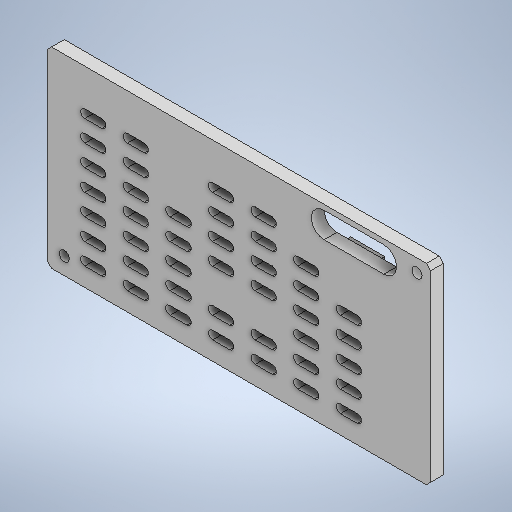
# Autodesk Inventor part: tampa final
Saved by Autodesk Inventor 2025 (Build 290162000, 162)
## iProperties
Created: 2026-04-08
Part Number: tampa final
Material: Genérico
Document SubType Name: Modeling
Designer: pedro
Density: 1 g/cm^3
Appearance: Padrão
Author: pedro
Autodesk Inventor part; units mm, degrees
ref_plane "YZ Plane" through (0, 0, 0) normal (1, 0, 0) x (0, 1, 0)
ref_plane "XZ Plane" through (0, 0, 0) normal (0, 1, 0) x (-1, 0, 0)
ref_plane "XY Plane" through (0, 0, 0) normal (0, 0, 1) x (1, 0, 0)
sketch "Esboço1" plane through (0, 0, 0) normal (0, 0, 1) x (1, 0, 0)
  line L0 (0, 0) -> (90, 0)
  line L1 (90, 0) -> (90, 45)
  line L2 (90, 45) -> (0, 45)
  line L3 (0, 45) -> (0, 0)
  dimension "d0" = 90
  dimension "d1" = 45
  constraints: 8 end point, 2 parallel, 1 horizontal, 1 perpendicular
  measures "d0" distance of L2.end L1.end
  measures "d1" distance of L1.end L0.end
extrude "Extrusão1" add sketch "Esboço1" along normal blind 3
sketch "Esboço3" plane through (0, 0, 3) normal (0, 0, 1) x (1, 0, 0)
  line L0 (0, 45) -> (0, 0) projected
  line L1 (90, 45) -> (0, 45) projected
  line L2 (63.8381, 29.7994) -> (75.2312, 29.7994)
  line L3 (8.8095, 35.3501) -> (12.8095, 35.3501) construction
  line L4 (8.8095, 34.3501) -> (12.8095, 34.3501)
  line L5 (12.8095, 36.3501) -> (8.8095, 36.3501)
  arc A0 (8.8095, 36.3501) -> (8.8095, 34.3501) centre (8.8095, 35.3501) ccw
  arc A1 (12.8095, 34.3501) -> (12.8095, 36.3501) centre (12.8095, 35.3501) ccw
  arc A2 (22.8095, 34.3501) -> (22.8095, 36.3501) centre (22.8095, 35.3501) ccw
  line L6 (18.8095, 35.3501) -> (22.8095, 35.3501) construction
  line L7 (18.8095, 34.3501) -> (22.8095, 34.3501)
  line L8 (22.8095, 36.3501) -> (18.8095, 36.3501)
  arc A3 (18.8095, 36.3501) -> (18.8095, 34.3501) centre (18.8095, 35.3501) ccw
  arc A4 (32.8095, 34.3501) -> (32.8095, 36.3501) centre (32.8095, 35.3501) ccw
  line L9 (28.8095, 35.3501) -> (32.8095, 35.3501) construction
  line L10 (28.8095, 34.3501) -> (32.8095, 34.3501)
  line L11 (32.8095, 36.3501) -> (28.8095, 36.3501)
  arc A5 (28.8095, 36.3501) -> (28.8095, 34.3501) centre (28.8095, 35.3501) ccw
  arc A6 (42.8095, 34.3501) -> (42.8095, 36.3501) centre (42.8095, 35.3501) ccw
  line L12 (38.8095, 35.3501) -> (42.8095, 35.3501) construction
  line L13 (38.8095, 34.3501) -> (42.8095, 34.3501)
  line L14 (42.8095, 36.3501) -> (38.8095, 36.3501)
  arc A7 (38.8095, 36.3501) -> (38.8095, 34.3501) centre (38.8095, 35.3501) ccw
  arc A8 (52.8095, 34.3501) -> (52.8095, 36.3501) centre (52.8095, 35.3501) ccw
  line L15 (48.8095, 35.3501) -> (52.8095, 35.3501) construction
  line L16 (48.8095, 34.3501) -> (52.8095, 34.3501)
  line L17 (52.8095, 36.3501) -> (48.8095, 36.3501)
  arc A9 (48.8095, 36.3501) -> (48.8095, 34.3501) centre (48.8095, 35.3501) ccw
  arc A10 (12.8095, 29.3501) -> (12.8095, 31.3501) centre (12.8095, 30.3501) ccw
  line L18 (8.8095, 30.3501) -> (12.8095, 30.3501) construction
  line L19 (8.8095, 29.3501) -> (12.8095, 29.3501)
  line L20 (12.8095, 31.3501) -> (8.8095, 31.3501)
  arc A11 (8.8095, 31.3501) -> (8.8095, 29.3501) centre (8.8095, 30.3501) ccw
  arc A12 (22.8095, 29.3501) -> (22.8095, 31.3501) centre (22.8095, 30.3501) ccw
  line L21 (18.8095, 30.3501) -> (22.8095, 30.3501) construction
  line L22 (18.8095, 29.3501) -> (22.8095, 29.3501)
  line L23 (22.8095, 31.3501) -> (18.8095, 31.3501)
  arc A13 (18.8095, 31.3501) -> (18.8095, 29.3501) centre (18.8095, 30.3501) ccw
  arc A14 (32.8095, 29.3501) -> (32.8095, 31.3501) centre (32.8095, 30.3501) ccw
  line L24 (28.8095, 30.3501) -> (32.8095, 30.3501) construction
  line L25 (28.8095, 29.3501) -> (32.8095, 29.3501)
  line L26 (32.8095, 31.3501) -> (28.8095, 31.3501)
  arc A15 (28.8095, 31.3501) -> (28.8095, 29.3501) centre (28.8095, 30.3501) ccw
  arc A16 (42.8095, 29.3501) -> (42.8095, 31.3501) centre (42.8095, 30.3501) ccw
  line L27 (38.8095, 30.3501) -> (42.8095, 30.3501) construction
  line L28 (38.8095, 29.3501) -> (42.8095, 29.3501)
  line L29 (42.8095, 31.3501) -> (38.8095, 31.3501)
  arc A17 (38.8095, 31.3501) -> (38.8095, 29.3501) centre (38.8095, 30.3501) ccw
  arc A18 (52.8095, 29.3501) -> (52.8095, 31.3501) centre (52.8095, 30.3501) ccw
  line L30 (48.8095, 30.3501) -> (52.8095, 30.3501) construction
  line L31 (48.8095, 29.3501) -> (52.8095, 29.3501)
  line L32 (52.8095, 31.3501) -> (48.8095, 31.3501)
  arc A19 (48.8095, 31.3501) -> (48.8095, 29.3501) centre (48.8095, 30.3501) ccw
  arc A20 (62.8095, 29.3501) -> (62.8095, 31.3501) centre (62.8095, 30.3501) ccw
  line L33 (58.8095, 30.3501) -> (62.8095, 30.3501) construction
  line L34 (58.8095, 29.3501) -> (62.8095, 29.3501)
  line L35 (62.8095, 31.3501) -> (58.8095, 31.3501)
  arc A21 (58.8095, 31.3501) -> (58.8095, 29.3501) centre (58.8095, 30.3501) ccw
  arc A22 (72.8095, 29.3501) -> (72.8095, 31.3501) centre (72.8095, 30.3501) ccw
  line L36 (68.8095, 30.3501) -> (72.8095, 30.3501) construction
  line L37 (68.8095, 29.3501) -> (72.8095, 29.3501)
  line L38 (72.8095, 31.3501) -> (68.8095, 31.3501)
  arc A23 (68.8095, 31.3501) -> (68.8095, 29.3501) centre (68.8095, 30.3501) ccw
  arc A24 (12.8095, 24.3501) -> (12.8095, 26.3501) centre (12.8095, 25.3501) ccw
  line L39 (8.8095, 25.3501) -> (12.8095, 25.3501) construction
  line L40 (8.8095, 24.3501) -> (12.8095, 24.3501)
  line L41 (12.8095, 26.3501) -> (8.8095, 26.3501)
  arc A25 (8.8095, 26.3501) -> (8.8095, 24.3501) centre (8.8095, 25.3501) ccw
  arc A26 (22.8095, 24.3501) -> (22.8095, 26.3501) centre (22.8095, 25.3501) ccw
  line L42 (18.8095, 25.3501) -> (22.8095, 25.3501) construction
  line L43 (18.8095, 24.3501) -> (22.8095, 24.3501)
  line L44 (22.8095, 26.3501) -> (18.8095, 26.3501)
  arc A27 (18.8095, 26.3501) -> (18.8095, 24.3501) centre (18.8095, 25.3501) ccw
  arc A28 (32.8095, 24.3501) -> (32.8095, 26.3501) centre (32.8095, 25.3501) ccw
  line L45 (28.8095, 25.3501) -> (32.8095, 25.3501) construction
  line L46 (28.8095, 24.3501) -> (32.8095, 24.3501)
  line L47 (32.8095, 26.3501) -> (28.8095, 26.3501)
  arc A29 (28.8095, 26.3501) -> (28.8095, 24.3501) centre (28.8095, 25.3501) ccw
  arc A30 (42.8095, 24.3501) -> (42.8095, 26.3501) centre (42.8095, 25.3501) ccw
  line L48 (38.8095, 25.3501) -> (42.8095, 25.3501) construction
  line L49 (38.8095, 24.3501) -> (42.8095, 24.3501)
  line L50 (42.8095, 26.3501) -> (38.8095, 26.3501)
  arc A31 (38.8095, 26.3501) -> (38.8095, 24.3501) centre (38.8095, 25.3501) ccw
  arc A32 (52.8095, 24.3501) -> (52.8095, 26.3501) centre (52.8095, 25.3501) ccw
  line L51 (48.8095, 25.3501) -> (52.8095, 25.3501) construction
  line L52 (48.8095, 24.3501) -> (52.8095, 24.3501)
  line L53 (52.8095, 26.3501) -> (48.8095, 26.3501)
  arc A33 (48.8095, 26.3501) -> (48.8095, 24.3501) centre (48.8095, 25.3501) ccw
  arc A34 (62.8095, 24.3501) -> (62.8095, 26.3501) centre (62.8095, 25.3501) ccw
  line L54 (58.8095, 25.3501) -> (62.8095, 25.3501) construction
  line L55 (58.8095, 24.3501) -> (62.8095, 24.3501)
  line L56 (62.8095, 26.3501) -> (58.8095, 26.3501)
  arc A35 (58.8095, 26.3501) -> (58.8095, 24.3501) centre (58.8095, 25.3501) ccw
  arc A36 (72.8095, 24.3501) -> (72.8095, 26.3501) centre (72.8095, 25.3501) ccw
  line L57 (68.8095, 25.3501) -> (72.8095, 25.3501) construction
  line L58 (68.8095, 24.3501) -> (72.8095, 24.3501)
  line L59 (72.8095, 26.3501) -> (68.8095, 26.3501)
  arc A37 (68.8095, 26.3501) -> (68.8095, 24.3501) centre (68.8095, 25.3501) ccw
  arc A38 (12.8095, 19.3501) -> (12.8095, 21.3501) centre (12.8095, 20.3501) ccw
  line L60 (8.8095, 20.3501) -> (12.8095, 20.3501) construction
  line L61 (8.8095, 19.3501) -> (12.8095, 19.3501)
  line L62 (12.8095, 21.3501) -> (8.8095, 21.3501)
  arc A39 (8.8095, 21.3501) -> (8.8095, 19.3501) centre (8.8095, 20.3501) ccw
  arc A40 (22.8095, 19.3501) -> (22.8095, 21.3501) centre (22.8095, 20.3501) ccw
  line L63 (18.8095, 20.3501) -> (22.8095, 20.3501) construction
  line L64 (18.8095, 19.3501) -> (22.8095, 19.3501)
  line L65 (22.8095, 21.3501) -> (18.8095, 21.3501)
  arc A41 (18.8095, 21.3501) -> (18.8095, 19.3501) centre (18.8095, 20.3501) ccw
  arc A42 (32.8095, 19.3501) -> (32.8095, 21.3501) centre (32.8095, 20.3501) ccw
  line L66 (28.8095, 20.3501) -> (32.8095, 20.3501) construction
  line L67 (28.8095, 19.3501) -> (32.8095, 19.3501)
  line L68 (32.8095, 21.3501) -> (28.8095, 21.3501)
  arc A43 (28.8095, 21.3501) -> (28.8095, 19.3501) centre (28.8095, 20.3501) ccw
  arc A44 (42.8095, 19.3501) -> (42.8095, 21.3501) centre (42.8095, 20.3501) ccw
  line L69 (38.8095, 20.3501) -> (42.8095, 20.3501) construction
  line L70 (38.8095, 19.3501) -> (42.8095, 19.3501)
  line L71 (42.8095, 21.3501) -> (38.8095, 21.3501)
  arc A45 (38.8095, 21.3501) -> (38.8095, 19.3501) centre (38.8095, 20.3501) ccw
  arc A46 (52.8095, 19.3501) -> (52.8095, 21.3501) centre (52.8095, 20.3501) ccw
  line L72 (48.8095, 20.3501) -> (52.8095, 20.3501) construction
  line L73 (48.8095, 19.3501) -> (52.8095, 19.3501)
  line L74 (52.8095, 21.3501) -> (48.8095, 21.3501)
  arc A47 (48.8095, 21.3501) -> (48.8095, 19.3501) centre (48.8095, 20.3501) ccw
  arc A48 (62.8095, 19.3501) -> (62.8095, 21.3501) centre (62.8095, 20.3501) ccw
  line L75 (58.8095, 20.3501) -> (62.8095, 20.3501) construction
  line L76 (58.8095, 19.3501) -> (62.8095, 19.3501)
  line L77 (62.8095, 21.3501) -> (58.8095, 21.3501)
  arc A49 (58.8095, 21.3501) -> (58.8095, 19.3501) centre (58.8095, 20.3501) ccw
  arc A50 (72.8095, 19.3501) -> (72.8095, 21.3501) centre (72.8095, 20.3501) ccw
  line L78 (68.8095, 20.3501) -> (72.8095, 20.3501) construction
  line L79 (68.8095, 19.3501) -> (72.8095, 19.3501)
  line L80 (72.8095, 21.3501) -> (68.8095, 21.3501)
  arc A51 (68.8095, 21.3501) -> (68.8095, 19.3501) centre (68.8095, 20.3501) ccw
  arc A52 (12.8095, 14.3501) -> (12.8095, 16.3501) centre (12.8095, 15.3501) ccw
  line L81 (8.8095, 15.3501) -> (12.8095, 15.3501) construction
  line L82 (8.8095, 14.3501) -> (12.8095, 14.3501)
  line L83 (12.8095, 16.3501) -> (8.8095, 16.3501)
  arc A53 (8.8095, 16.3501) -> (8.8095, 14.3501) centre (8.8095, 15.3501) ccw
  arc A54 (22.8095, 14.3501) -> (22.8095, 16.3501) centre (22.8095, 15.3501) ccw
  line L84 (18.8095, 15.3501) -> (22.8095, 15.3501) construction
  line L85 (18.8095, 14.3501) -> (22.8095, 14.3501)
  line L86 (22.8095, 16.3501) -> (18.8095, 16.3501)
  arc A55 (18.8095, 16.3501) -> (18.8095, 14.3501) centre (18.8095, 15.3501) ccw
  arc A56 (32.8095, 14.3501) -> (32.8095, 16.3501) centre (32.8095, 15.3501) ccw
  line L87 (28.8095, 15.3501) -> (32.8095, 15.3501) construction
  line L88 (28.8095, 14.3501) -> (32.8095, 14.3501)
  line L89 (32.8095, 16.3501) -> (28.8095, 16.3501)
  arc A57 (28.8095, 16.3501) -> (28.8095, 14.3501) centre (28.8095, 15.3501) ccw
  arc A58 (42.8095, 14.3501) -> (42.8095, 16.3501) centre (42.8095, 15.3501) ccw
  line L90 (38.8095, 15.3501) -> (42.8095, 15.3501) construction
  line L91 (38.8095, 14.3501) -> (42.8095, 14.3501)
  line L92 (42.8095, 16.3501) -> (38.8095, 16.3501)
  arc A59 (38.8095, 16.3501) -> (38.8095, 14.3501) centre (38.8095, 15.3501) ccw
  arc A60 (52.8095, 14.3501) -> (52.8095, 16.3501) centre (52.8095, 15.3501) ccw
  line L93 (48.8095, 15.3501) -> (52.8095, 15.3501) construction
  line L94 (48.8095, 14.3501) -> (52.8095, 14.3501)
  line L95 (52.8095, 16.3501) -> (48.8095, 16.3501)
  arc A61 (48.8095, 16.3501) -> (48.8095, 14.3501) centre (48.8095, 15.3501) ccw
  arc A62 (62.8095, 14.3501) -> (62.8095, 16.3501) centre (62.8095, 15.3501) ccw
  line L96 (58.8095, 15.3501) -> (62.8095, 15.3501) construction
  line L97 (58.8095, 14.3501) -> (62.8095, 14.3501)
  line L98 (62.8095, 16.3501) -> (58.8095, 16.3501)
  arc A63 (58.8095, 16.3501) -> (58.8095, 14.3501) centre (58.8095, 15.3501) ccw
  arc A64 (72.8095, 14.3501) -> (72.8095, 16.3501) centre (72.8095, 15.3501) ccw
  line L99 (68.8095, 15.3501) -> (72.8095, 15.3501) construction
  line L100 (68.8095, 14.3501) -> (72.8095, 14.3501)
  line L101 (72.8095, 16.3501) -> (68.8095, 16.3501)
  arc A65 (68.8095, 16.3501) -> (68.8095, 14.3501) centre (68.8095, 15.3501) ccw
  arc A66 (12.8095, 9.3501) -> (12.8095, 11.3501) centre (12.8095, 10.3501) ccw
  line L102 (8.8095, 10.3501) -> (12.8095, 10.3501) construction
  line L103 (8.8095, 9.3501) -> (12.8095, 9.3501)
  line L104 (12.8095, 11.3501) -> (8.8095, 11.3501)
  arc A67 (8.8095, 11.3501) -> (8.8095, 9.3501) centre (8.8095, 10.3501) ccw
  arc A68 (22.8095, 9.3501) -> (22.8095, 11.3501) centre (22.8095, 10.3501) ccw
  line L105 (18.8095, 10.3501) -> (22.8095, 10.3501) construction
  line L106 (18.8095, 9.3501) -> (22.8095, 9.3501)
  line L107 (22.8095, 11.3501) -> (18.8095, 11.3501)
  arc A69 (18.8095, 11.3501) -> (18.8095, 9.3501) centre (18.8095, 10.3501) ccw
  arc A70 (32.8095, 9.3501) -> (32.8095, 11.3501) centre (32.8095, 10.3501) ccw
  line L108 (28.8095, 10.3501) -> (32.8095, 10.3501) construction
  line L109 (28.8095, 9.3501) -> (32.8095, 9.3501)
  line L110 (32.8095, 11.3501) -> (28.8095, 11.3501)
  arc A71 (28.8095, 11.3501) -> (28.8095, 9.3501) centre (28.8095, 10.3501) ccw
  arc A72 (42.8095, 9.3501) -> (42.8095, 11.3501) centre (42.8095, 10.3501) ccw
  line L111 (38.8095, 10.3501) -> (42.8095, 10.3501) construction
  line L112 (38.8095, 9.3501) -> (42.8095, 9.3501)
  line L113 (42.8095, 11.3501) -> (38.8095, 11.3501)
  arc A73 (38.8095, 11.3501) -> (38.8095, 9.3501) centre (38.8095, 10.3501) ccw
  arc A74 (52.8095, 9.3501) -> (52.8095, 11.3501) centre (52.8095, 10.3501) ccw
  line L114 (48.8095, 10.3501) -> (52.8095, 10.3501) construction
  line L115 (48.8095, 9.3501) -> (52.8095, 9.3501)
  line L116 (52.8095, 11.3501) -> (48.8095, 11.3501)
  arc A75 (48.8095, 11.3501) -> (48.8095, 9.3501) centre (48.8095, 10.3501) ccw
  arc A76 (62.8095, 9.3501) -> (62.8095, 11.3501) centre (62.8095, 10.3501) ccw
  line L117 (58.8095, 10.3501) -> (62.8095, 10.3501) construction
  line L118 (58.8095, 9.3501) -> (62.8095, 9.3501)
  line L119 (62.8095, 11.3501) -> (58.8095, 11.3501)
  arc A77 (58.8095, 11.3501) -> (58.8095, 9.3501) centre (58.8095, 10.3501) ccw
  arc A78 (72.8095, 9.3501) -> (72.8095, 11.3501) centre (72.8095, 10.3501) ccw
  line L120 (68.8095, 10.3501) -> (72.8095, 10.3501) construction
  line L121 (68.8095, 9.3501) -> (72.8095, 9.3501)
  line L122 (72.8095, 11.3501) -> (68.8095, 11.3501)
  arc A79 (68.8095, 11.3501) -> (68.8095, 9.3501) centre (68.8095, 10.3501) ccw
  arc A80 (12.8095, 4.3501) -> (12.8095, 6.3501) centre (12.8095, 5.3501) ccw
  line L123 (8.8095, 5.3501) -> (13.3095, 5.3501) construction
  line L124 (8.8095, 4.3501) -> (12.8095, 4.3501)
  line L125 (12.8095, 6.3501) -> (8.8095, 6.3501)
  arc A81 (8.8095, 6.3501) -> (8.8095, 4.3501) centre (8.8095, 5.3501) ccw
  arc A82 (22.8095, 4.3501) -> (22.8095, 6.3501) centre (22.8095, 5.3501) ccw
  line L126 (18.8095, 5.3501) -> (23.3095, 5.3501) construction
  line L127 (18.8095, 4.3501) -> (22.8095, 4.3501)
  line L128 (22.8095, 6.3501) -> (18.8095, 6.3501)
  arc A83 (18.8095, 6.3501) -> (18.8095, 4.3501) centre (18.8095, 5.3501) ccw
  arc A84 (32.8095, 4.3501) -> (32.8095, 6.3501) centre (32.8095, 5.3501) ccw
  line L129 (28.8095, 5.3501) -> (32.8095, 5.3501) construction
  line L130 (28.8095, 4.3501) -> (32.8095, 4.3501)
  line L131 (32.8095, 6.3501) -> (28.8095, 6.3501)
  arc A85 (28.8095, 6.3501) -> (28.8095, 4.3501) centre (28.8095, 5.3501) ccw
  arc A86 (42.8095, 4.3501) -> (42.8095, 6.3501) centre (42.8095, 5.3501) ccw
  line L132 (38.8095, 5.3501) -> (42.8095, 5.3501) construction
  line L133 (38.8095, 4.3501) -> (42.8095, 4.3501)
  line L134 (42.8095, 6.3501) -> (38.8095, 6.3501)
  arc A87 (38.8095, 6.3501) -> (38.8095, 4.3501) centre (38.8095, 5.3501) ccw
  arc A88 (52.8095, 4.3501) -> (52.8095, 6.3501) centre (52.8095, 5.3501) ccw
  line L135 (48.8095, 5.3501) -> (52.8095, 5.3501) construction
  line L136 (48.8095, 4.3501) -> (52.8095, 4.3501)
  line L137 (52.8095, 6.3501) -> (48.8095, 6.3501)
  arc A89 (48.8095, 6.3501) -> (48.8095, 4.3501) centre (48.8095, 5.3501) ccw
  arc A90 (62.8095, 4.3501) -> (62.8095, 6.3501) centre (62.8095, 5.3501) ccw
  line L138 (58.8095, 5.3501) -> (62.8095, 5.3501) construction
  line L139 (58.8095, 4.3501) -> (62.8095, 4.3501)
  line L140 (62.8095, 6.3501) -> (58.8095, 6.3501)
  arc A91 (58.8095, 6.3501) -> (58.8095, 4.3501) centre (58.8095, 5.3501) ccw
  arc A92 (72.8095, 4.3501) -> (72.8095, 6.3501) centre (72.8095, 5.3501) ccw
  line L141 (68.8095, 5.3501) -> (72.8095, 5.3501) construction
  line L142 (68.8095, 4.3501) -> (72.8095, 4.3501)
  line L143 (72.8095, 6.3501) -> (68.8095, 6.3501)
  arc A93 (68.8095, 6.3501) -> (68.8095, 4.3501) centre (68.8095, 5.3501) ccw
  point P0 (0, 23.5)
  point P1 (48.3095, 21.3501)
  point P2 (10.8095, 35.3501)
  point P3 (20.8095, 35.3501)
  point P4 (30.8095, 35.3501)
  point P5 (40.8095, 35.3501)
  point P6 (50.8095, 35.3501)
  point P7 (10.8095, 30.3501)
  point P8 (20.8095, 30.3501)
  point P9 (30.8095, 30.3501)
  point P10 (40.8095, 30.3501)
  point P11 (50.8095, 30.3501)
  point P12 (60.8095, 30.3501)
  point P13 (70.8095, 30.3501)
  point P14 (10.8095, 25.3501)
  point P15 (20.8095, 25.3501)
  point P16 (30.8095, 25.3501)
  point P17 (40.8095, 25.3501)
  point P18 (50.8095, 25.3501)
  point P19 (60.8095, 25.3501)
  point P20 (70.8095, 25.3501)
  point P21 (10.8095, 20.3501)
  point P22 (20.8095, 20.3501)
  point P23 (30.8095, 20.3501)
  point P24 (40.8095, 20.3501)
  point P25 (50.8095, 20.3501)
  point P26 (60.8095, 20.3501)
  point P27 (70.8095, 20.3501)
  point P28 (10.8095, 15.3501)
  point P29 (20.8095, 15.3501)
  point P30 (30.8095, 15.3501)
  point P31 (40.8095, 15.3501)
  point P32 (50.8095, 15.3501)
  point P33 (60.8095, 15.3501)
  point P34 (70.8095, 15.3501)
  point P35 (10.8095, 10.3501)
  point P36 (20.8095, 10.3501)
  point P37 (30.8095, 10.3501)
  point P38 (40.8095, 10.3501)
  point P39 (50.8095, 10.3501)
  point P40 (60.8095, 10.3501)
  point P41 (70.8095, 10.3501)
  point P42 (10.8095, 5.3501)
  point P43 (20.8095, 5.3501)
  point P44 (30.8095, 5.3501)
  point P45 (40.8095, 5.3501)
  point P46 (50.8095, 5.3501)
  point P47 (60.8095, 5.3501)
  point P48 (70.8095, 5.3501)
  dimension "d42" = 4
  dimension "d43" = 2
  dimension "d44" = 10
  dimension "d45" = 5
  constraints: 376 end point, 188 point on circle, 94 centre point, 4 tangent, 2 horizontal, 2 point on line, 1 midpoint, 1 parallel
  measures "d42" distance of L3.start L3.end
  measures "d43" diameter of A1
  measures "d44" distance of L3.end L6.end
  measures "d45" distance of L3.end L18.end
extrude "Extrusão3" cut sketch "Esboço3" against normal blind 4 contours A0 L5 A1 L4 | L7 A3 L8 A2 | L13 A7 L14 A6 | L16 A9 L17 A8 | L19 A11 L20 A10 | L22 A13 L23 A12 | L28 A17 L29 A16 | L31 A19 L32 A18 | L34 A21 L35 A20 | L40 A25 L41 A24 | L43 A27 L44 A26 | L46 A29 L47 A28 | L49 A31 L50 A30 | L52 A33 L53 A32 | L55 A35 L56 A34 | L58 A37 L59 A36 | L61 A39 L62 A38 | L64 A41 L65 A40 | L67 A43 L68 A42 | L70 A45 L71 A44 | L73 A47 L74 A46 | L76 A49 L77 A48 | L79 A51 L80 A50 | L82 A53 L83 A52 | L85 A55 L86 A54 | L88 A57 L89 A56 | L97 A63 L98 A62 | L100 A65 L101 A64 | L103 A67 L104 A66 | L106 A69 L107 A68 | L109 A71 L110 A70 | L112 A73 L113 A72 | L115 A75 L116 A74 | L118 A77 L119 A76 | L121 A79 L122 A78 | L124 A81 L125 A80 | L127 A83 L128 A82 | L130 A85 L131 A84 | L133 A87 L134 A86 | L136 A89 L137 A88 | L139 A91 L140 A90 | L142 A93 L143 A92
sketch "Esboço4" plane through (0, 0, 3) normal (0, 0, 1) x (1, 0, 0)
  line L0 (2, 2) -> (6, 2)
  line L1 (6, 2) -> (6, 6)
  line L2 (6, 6) -> (2, 6)
  line L3 (2, 6) -> (2, 2)
  line L4 (0, 45) -> (0, 0) projected
  line L5 (0, 0) -> (90, 0) projected
  line L6 (88.8, 43.959) -> (84.8, 43.959)
  line L7 (84.8, 43.959) -> (84.8, 39.959)
  line L8 (84.8, 39.959) -> (88.8, 39.959)
  line L9 (88.8, 39.959) -> (88.8, 43.959)
  line L10 (90, 45) -> (0, 45) projected
  line L11 (90, 0) -> (90, 45) projected
  circle A0 centre (86.8, 41.959) radius 1.2
  circle A1 centre (4, 4) radius 1.2
  point P0 (0, 21.5)
  point P1 (90, 23.5)
  point P2 (88.8, 41.959)
  point P3 (86.8, 43.959)
  point P4 (4, 6)
  point P5 (2, 4)
  dimension "d20" = 4
  dimension "d21" = 4
  dimension "d24" = 4
  dimension "d25" = 4
  dimension "d28" = 2.4
  dimension "d29" = 2.4
  dimension "d46" = 3.041
  dimension "d47" = 3.2
  dimension "d48" = 4
  dimension "d49" = 4
  constraints: 16 end point, 4 midpoint, 4 parallel, 2 centre point, 2 horizontal, 2 horizontal alignment, 2 perpendicular, 2 vertical alignment
  measures "d20" distance of L2.end L1.end
  measures "d21" distance of L1.end L0.end
  measures "d24" distance of L8.end L7.end
  measures "d25" distance of L7.end L6.end
  measures "d28" diameter of A0
  measures "d29" diameter of A1
  measures "d46" distance from line of L10 A0.centre
  measures "d47" distance from line of L11 A0.centre
  measures "d48" distance from line of L4 A1.centre
  measures "d49" distance from line of L5 A1.centre
extrude "Extrusão4" cut sketch "Esboço4" against normal blind 4 contours A0 | A1
sketch "Esboço5" plane through (0, 0, 3) normal (0, 0, 1) x (1, 0, 0)
  line L0 (62, 40.8) -> (82, 40.8) construction
  line L1 (65, 37.8) -> (79, 37.8)
  line L2 (79, 43.8) -> (65, 43.8)
  arc A0 (65, 43.8) -> (65, 37.8) centre (65, 40.8) ccw
  arc A1 (79, 37.8) -> (79, 43.8) centre (79, 40.8) ccw
  line L3 (90, 45) -> (0, 45) projected
  line L4 (90, 0) -> (90, 45) projected
  point P0 (0, 0)
  point P1 (72, 40.8)
  point P2 (82, 40.8)
  point P3 (62, 40.8)
  point P4 (90, 23.5)
  dimension "d32" = 20
  dimension "d33" = 6
  dimension "d34" = 1.2
  dimension "d36" = 28
  constraints: 8 end point, 8 point on circle, 4 tangent, 2 centre point, 2 point on line, 1 horizontal, 1 midpoint, 1 parallel
  measures "d32" distance of point (82, 40.8) point (62, 40.8)
  measures "d33" distance between parallel lines of L1 L2
  measures "d34" distance between parallel lines of L2 L3
  measures "d36" distance from line of L4 L0.start
extrude "Extrusão5" cut sketch "Esboço5" against normal blind 4
chamfer "Chanfro1" distance 1 angle 45 4 edges at (0, 45, 1.5) (90, 45, 1.5) (90, 0, 1.5) (0, 0, 1.5)
sketch "Esboço6" plane through (0, 0, 0) normal (0, 0, -1) x (-1, 0, 0)
  line L0 (-50.9434, 13) -> (-42.9434, 13)
  line L1 (-42.9434, 13) -> (-42.9434, 16)
  line L2 (-42.9434, 16) -> (-50.9434, 16)
  line L3 (-50.9434, 16) -> (-50.9434, 13)
  line L4 (-1, 0) -> (-89, 0) projected
  line L5 (-50.3101, 22.8) -> (-42.3101, 22.8)
  line L6 (-42.3101, 22.8) -> (-42.3101, 24.3)
  line L7 (-42.3101, 24.3) -> (-50.3101, 24.3)
  line L8 (-50.3101, 24.3) -> (-50.3101, 22.8)
  line L9 (-89, 45) -> (-1, 45) projected
  line L10 (-71.2, 32) -> (-63.2, 32)
  line L11 (-63.2, 32) -> (-63.2, 33.5)
  line L12 (-63.2, 33.5) -> (-71.2, 33.5)
  line L13 (-71.2, 33.5) -> (-71.2, 32)
  line L14 (-33.2, 32) -> (-25.2, 32)
  line L15 (-25.2, 32) -> (-25.2, 33.5)
  line L16 (-25.2, 33.5) -> (-33.2, 33.5)
  line L17 (-33.2, 33.5) -> (-33.2, 32)
  line L18 (-90, 1) -> (-90, 44) projected
  point P0 (0, 0)
  point P1 (-46.9434, 16)
  point P2 (-44.5745, 32.0802)
  point P3 (-46.3101, 24.3)
  point P4 (-73.5012, 29.8757)
  point P5 (-67.2, 33.5)
  point P6 (-29.2, 33.5)
  point P7 (-33.2, 32.75)
  point P8 (-63.2, 32.75)
  dimension "d50" = 8
  dimension "d51" = 3
  dimension "d52" = 13
  dimension "d57" = 8
  dimension "d58" = 1.5
  dimension "d59" = 20.7
  dimension "d60" = 8
  dimension "d61" = 1.5
  dimension "d62" = 8
  dimension "d63" = 1.5
  dimension "d64" = 11.5
  dimension "d65" = 18.8
  dimension "d66" = 38
  constraints: 32 end point, 7 parallel, 6 midpoint, 4 horizontal, 4 perpendicular, 1 horizontal alignment
  measures "d50" distance of L2.end L1.end
  measures "d51" distance of L1.end L1.start
  measures "d52" distance between parallel lines of L4 L0
  measures "d57" distance of L7.end L6.end
  measures "d58" distance of L6.end L5.end
  measures "d59" distance between parallel lines of L7 L9
  measures "d60" distance of L13.start L11.end
  measures "d61" distance of L11.end L11.start
  measures "d62" distance of L17.start L16.start
  measures "d63" distance of L16.start L15.start
  measures "d64" distance between parallel lines of L9 L12
  measures "d65" distance between parallel lines of L18 L13
  measures "d66" distance between parallel lines of L13 L17
extrude "Extrusão6" add sketch "Esboço6" along normal blind 5 and the other way blind 2 contours L3 L2 L1 L0 | L8 L7 L6 L5
extrude "Extrusão7" add sketch "Esboço6" along normal blind 5 and the other way blind 2 contours L13 L12 L11 L10 | L17 L16 L15 L14
